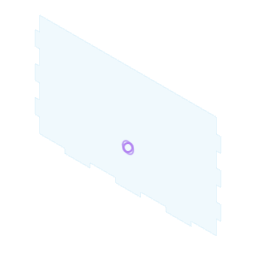
Box for nanoboard (Autodesk Fusion 360 design; units mm, degrees)
Autodesk Fusion 360 part; units mm, degrees
note: some values were not read from the file. Set by a fixed rule: which sketch regions a step uses.
(part 1 of 2)
sketch "Sketch1" plane through (0, 0, 0) normal (0, 1, 0) x (1, 0, 0) in component "Back"
  line L0 (0, 0) -> (126.286, 0)
  line L1 (126.286, 0) -> (126.286, -73)
  line L2 (126.286, -73) -> (0, -73)
  line L3 (0, -73) -> (0, 0)
  line L4 (3, -73) -> (3, 0)
  line L5 (0, -13) -> (3, -13)
  line L6 (0, -23) -> (3, -23)
  line L7 (3, -35) -> (3, -33)
  line L8 (3, -33) -> (0, -33)
  line L9 (0, -33) -> (0, -36.5)
  line L10 (0, -63) -> (3, -63)
  line L11 (3, -63) -> (3, -53)
  line L12 (3, -53) -> (0, -53)
  line L13 (0, -53) -> (0, -63)
  line L14 (0, -43) -> (3, -43)
  line L15 (63.143, -73) -> (63.143, 0) construction
  line L16 (126.286, -63) -> (123.286, -63)
  line L17 (123.286, -53) -> (126.286, -53)
  line L18 (123.286, -73) -> (123.286, 0)
  line L19 (126.286, -43) -> (123.286, -43)
  line L20 (123.286, -33) -> (126.286, -33)
  line L21 (126.286, -23) -> (123.286, -23)
  line L22 (126.286, -13) -> (123.286, -13)
  line L23 (126.286, -3) -> (0, -3)
  line L24 (106.1023, -3) -> (88.9186, -3)
  line L25 (88.9186, -3) -> (88.9186, 0)
  line L26 (88.9186, 0) -> (106.1023, 0)
  line L27 (106.1023, 0) -> (106.1023, -3)
  line L28 (71.7349, -3) -> (54.5511, -3)
  line L29 (54.5511, -3) -> (54.5511, 0)
  line L30 (54.5511, 0) -> (71.7349, 0)
  line L31 (71.7349, 0) -> (71.7349, -3)
  line L32 (37.3674, -3) -> (0, -3)
  line L33 (0, -3) -> (0, 0)
  line L34 (0, 0) -> (37.3674, 0)
  line L35 (37.3674, 0) -> (37.3674, -3)
  line L36 (126.286, -73) -> (0, -73)
  line L37 (0, -73) -> (0, -76)
  line L38 (0, -76) -> (126.286, -76)
  line L39 (126.286, -76) -> (126.286, -73)
  line L40 (123.286, -73) -> (123.286, -76)
  line L41 (3, -73) -> (3, -76)
  line L42 (20.1837, -3) -> (20.1837, 0)
  dimension "d10" = 3
  dimension "d58" = 3
  dimension "d137" = 3
  dimension "d171" = 70
  dimension "d172" = 120.286
  dimension "d173" = 17.1837
  dimension "d174" = 17.1837
  dimension "d175" = 17.1837
  dimension "d176" = 17.1837
  dimension "d177" = 17.1837
  dimension "d178" = 17.1837
  dimension "d179" = 22.8571
  dimension "d188" = 10
  dimension "d189" = 10
  dimension "d190" = 10
  dimension "d191" = 10
  dimension "d192" = 10
  dimension "d193" = 10
  dimension "d194" = 10
  constraint horizontal L0
  constraint vertical L1
  constraint horizontal L2
  constraint vertical L3
  constraint coincident L0.start L3.end
  constraint coincident L2 L4.start
  constraint coincident L0 L4.end
  constraint perpendicular L0 L4
  constraint coincident L3 L5.start
  constraint coincident L4 L5.end
  constraint perpendicular L4 L5
  constraint coincident L3 L6.start
  constraint coincident L4 L6.end
  constraint perpendicular L4 L6
  constraint vertical L7
  constraint horizontal L8
  constraint vertical L9
  constraint coincident L4 L7.end
  constraint midpoint L3 L9.end
  constraint horizontal L10
  constraint vertical L11
  constraint horizontal L12
  constraint vertical L13
  constraint coincident L4 L11.end
  constraint coincident L3 L10.start
  constraint coincident L3 L14.start
  constraint coincident L4 L14.end
  constraint perpendicular L4 L14
  constraint midpoint L2 L15.start
  constraint midpoint L0 L15.end
  constraint symmetric L4.start L15 L18.start
  constraint symmetric L4.end L15 L18.end
  constraint symmetric L5.start L15 L22.start
  constraint symmetric L5.end L15 L22.end
  constraint symmetric L6.start L15 L21.start
  constraint symmetric L6.end L15 L21.end
  constraint symmetric L7.end L15 L20.start
  constraint symmetric L8.end L15 L20.end
  constraint symmetric L10.start L15 L16.start
  constraint symmetric L10.end L15 L16.end
  constraint symmetric L11.end L15 L17.start
  constraint symmetric L12.end L15 L17.end
  constraint symmetric L14.start L15 L19.start
  constraint symmetric L14.end L15 L19.end
  constraint coincident L1 L23.start
  constraint coincident L3 L23.end
  constraint perpendicular L4 L23
  constraint horizontal L24
  constraint vertical L25
  constraint horizontal L26
  constraint vertical L27
  constraint coincident L0 L25.end
  constraint coincident L23 L24.start
  constraint horizontal L28
  constraint vertical L29
  constraint horizontal L30
  constraint vertical L31
  constraint coincident L23 L28.start
  constraint horizontal L32
  constraint vertical L33
  constraint horizontal L34
  constraint vertical L35
  constraint coincident L0 L3.end
  constraint coincident L23 L32.start
  constraint horizontal L36
  constraint vertical L37
  constraint horizontal L38
  constraint vertical L39
  constraint coincident L38 L40.end
  constraint perpendicular L36 L40
  constraint coincident L38 L41.end
  constraint perpendicular L38 L41
  constraint coincident L32 L42.start
  constraint coincident L34 L42.end
  constraint perpendicular L34 L42
  measures "d10" distance of L3 L4
  measures "d58" distance of L0 L23
  measures "d137" distance of L36 L38
  measures "d171" distance of L23 L36
  measures "d172" distance of L4 L18
  measures "d173" distance of L18 L27
  measures "d174" distance of L25 L27
  measures "d175" distance of L25 L31
  measures "d176" distance of L29 L31
  measures "d177" distance of L29 L35
  measures "d178" distance of L35 L42
  measures "d188" distance of L2 L10
  measures "d189" distance of L10 L12
  measures "d190" distance of L12 L14
  measures "d191" distance of L8 L14
  measures "d192" distance of L6 L8
  measures "d193" distance of L5 L6
  measures "d194" distance of L5 L23
extrude "Extrude1" add sketch "Sketch1" against normal blind 3 contours L0 L23 L32 L34 L35 L42 | L2 L4 L7 L11 L18 L23 L24 L28 L32 L36 | L3 L4 L5 L6 | L0 L23 L28 L29 L30 L31 | L3 L4 L7 L8 L9 L14 | L0 L23 L24 L25 L26 L27 | L3 L4 L10 L11 L12 L13 | L1 L18 L21 L22 | L2 L36 L38 L40 L41 | L1 L18 L19 L20 | L1 L16 L17 L18 makes body 1 in component "Back"
sketch "Sketch1 (2)" plane through (0, 0, 0) normal (1, 0, 0) x (0, 1, 0) in component "left"
  line L0 (0, 0) -> (-86, 0)
  line L1 (-86, 0) -> (-86, 73)
  line L2 (-86, 73) -> (0, 73)
  line L3 (0, 73) -> (0, 0)
  line L4 (0, 3) -> (-86, 3)
  line L5 (-19, 3) -> (-35, 3)
  line L6 (-35, 3) -> (-35, 0)
  line L7 (-35, 0) -> (-19, 0)
  line L8 (-19, 0) -> (-19, 3)
  line L9 (-48, 3) -> (-35, 3)
  line L10 (-43, 0) -> (-48, 0)
  line L11 (-51, 3) -> (-67, 3)
  line L12 (-67, 3) -> (-67, 0)
  line L13 (-67, 0) -> (-51, 0)
  line L14 (-51, 0) -> (-51, 3)
  line L15 (-3, 73) -> (-3, 0)
  circle A0 centre (-7.7793, 74.469) radius 5
  circle A1 centre (-7.7793, 74.469) radius 2.5
  line L16 (-43, 73) -> (-43, 0) construction
  line L17 (-83, 73) -> (-83, 0)
  line L18 (-86, 63) -> (-83, 63)
  line L19 (-83, 63) -> (-83, 31.2457)
  line L20 (-86, 31.2457) -> (-86, 63)
  line L21 (-86, 53) -> (-83, 53)
  line L22 (-83, 53) -> (-83, 43)
  line L23 (-83, 43) -> (-86, 43)
  line L24 (-86, 43) -> (-86, 53)
  line L25 (-83, 20) -> (-83, 33)
  line L26 (-83, 33) -> (-86, 33)
  line L27 (-86, 33) -> (-86, 36.5)
  line L28 (-86, 23) -> (-83, 23)
  line L29 (-83, 23) -> (-83, 13)
  line L30 (-83, 13) -> (-86, 13)
  line L31 (-86, 13) -> (-86, 23)
  line L32 (0, 63) -> (-3, 63)
  line L33 (0, 53) -> (-3, 53)
  line L34 (-3, 43) -> (0, 43)
  line L35 (-3, 33) -> (0, 33)
  line L36 (0, 23) -> (-3, 23)
  line L37 (-3, 13) -> (0, 13)
  line L38 (-86, 73) -> (0, 73)
  line L39 (0, 73) -> (0, 76)
  line L40 (0, 76) -> (-86, 76)
  line L41 (-86, 76) -> (-86, 73)
  circle A2 centre (-43, 7.9695) radius 5
  dimension "d67" = 3
  dimension "d111" = 3
  dimension "d112" = 10
  dimension "d113" = 5
  dimension "d161" = 3
  dimension "d162" = 10
  dimension "d166" = 10
  dimension "d167" = 10
  dimension "d169" = 3
  dimension "d180" = 16
  dimension "d181" = 16
  dimension "d182" = 16
  dimension "d183" = 16
  dimension "d185" = 80
  dimension "d186" = 16
  dimension "d195" = 70
  dimension "d196" = 10
  dimension "d197" = 10
  dimension "d198" = 10
  dimension "d199" = 10
  dimension "d233" = 10
  constraint horizontal L0
  constraint vertical L1
  constraint horizontal L2
  constraint vertical L3
  constraint coincident L0.start L3.end
  constraint coincident L3 L4.start
  constraint coincident L1 L4.end
  constraint perpendicular L1 L4
  constraint horizontal L5
  constraint vertical L6
  constraint horizontal L7
  constraint vertical L8
  constraint coincident L0 L6.end
  constraint coincident L4 L5.start
  constraint horizontal L9
  constraint horizontal L10
  constraint midpoint L0 L10.start
  constraint coincident L4 L9.start
  constraint horizontal L11
  constraint vertical L12
  constraint horizontal L13
  constraint vertical L14
  constraint coincident L0 L12.end
  constraint coincident L4 L11.start
  constraint coincident L2 L15.start
  constraint coincident L0 L15.end
  constraint perpendicular L0 L15
  constraint coincident L15.start A0
  constraint concentric A0 A1
  constraint midpoint L2 L16.start
  constraint coincident L2 L17.start
  constraint coincident L0 L17.end
  constraint perpendicular L0 L17
  constraint horizontal L18
  constraint vertical L19
  constraint vertical L20
  constraint coincident L17 L19.end
  constraint coincident L1 L18.start
  constraint horizontal L21
  constraint vertical L22
  constraint horizontal L23
  constraint vertical L24
  constraint coincident L17 L22.end
  constraint coincident L1 L21.start
  constraint vertical L25
  constraint horizontal L26
  constraint vertical L27
  constraint coincident L17 L25.end
  constraint midpoint L1 L27.end
  constraint horizontal L28
  constraint vertical L29
  constraint horizontal L30
  constraint vertical L31
  constraint coincident L17 L29.end
  constraint coincident L1 L28.start
  constraint symmetric L16 L18.start L32.start
  constraint symmetric L16 L18.end L32.end
  constraint symmetric L16 L21.start L33.start
  constraint symmetric L16 L21.end L33.end
  constraint symmetric L16 L22.end L34.start
  constraint symmetric L16 L23.end L34.end
  constraint symmetric L16 L25.end L35.start
  constraint symmetric L16 L26.end L35.end
  constraint symmetric L16 L28.start L36.start
  constraint symmetric L16 L28.end L36.end
  constraint symmetric L16 L29.end L37.start
  constraint symmetric L16 L30.end L37.end
  constraint horizontal L38
  constraint vertical L39
  constraint horizontal L40
  constraint vertical L41
  constraint coincident L16 A2.centre
  measures "d67" distance of L0 L4
  measures "d111" distance of L3 L15
  measures "d112" diameter of A0
  measures "d113" diameter of A1
  measures "d161" distance of L1 L17
  measures "d162" distance of L2 L18
  measures "d166" distance of L18 L21
  measures "d167" distance of L21 L23
  measures "d169" distance of L38 L40
  measures "d180" distance of L8 L15
  measures "d181" distance of L6 L8
  measures "d182" distance of L6 L14
  measures "d183" distance of L12 L14
  measures "d185" distance of L15 L17
  measures "d186" distance of L12 L17
  measures "d195" distance of L2 L4
  measures "d196" distance of L23 L26
  measures "d197" distance of L26 L28
  measures "d198" distance of L28 L30
  measures "d199" distance of L4 L30
  measures "d233" diameter of A2
extrude "Extrude1'" add sketch "Sketch1 (2)" along normal blind 3 separate body contours L3 L4 L15 L37 | L0 L4 L5 L6 L7 L8 | L2 L4 L5 L9 L11 L15 A0 L17 L19 L22 L25 L29 L38 A2 | L3 L15 L35 L36 | L3 L15 L33 L34 | L0 L4 L11 L12 L13 L14 | L2 L3 L15 L32 L38 | L1 L4 L17 L30 | L2 A0 A1 L38 | L2 A0 A1 L38 L40 | L2 A0 A1 L38 L40 | L2 A0 L38 L40 L41 | A0 A1 L40 | L1 L2 L17 L18 L38 | L1 L17 L19 L20 L25 L26 L28 | L1 L17 L19 L20 L21 L22 L23 L24 makes body 2 in component "left"
ref_plane "WorkPlane3" through (63.143, -43, 38) normal (0, 1, 0) x (1, 0, 0)
sketch "Sketch2" plane through (32.5, -43, 21.5) normal (0, 1, 0) x (1, 0, 0) in component "Front"
  line L0 (0, 0) -> (126.286, 0)
  line L1 (126.286, 0) -> (126.286, -73)
  line L2 (126.286, -73) -> (0, -73)
  line L3 (0, -73) -> (0, 0)
  line L4 (3, -73) -> (3, 0)
  line L5 (0, -3) -> (126.286, -3)
  line L6 (123.286, -73) -> (123.286, 0)
  line L7 (0, -73) -> (3, -73)
  line L8 (3, -73) -> (3, -63)
  line L9 (3, -63) -> (0, -63)
  line L10 (0, -63) -> (0, -73)
  line L11 (0, -53) -> (3, -53)
  line L12 (3, -53) -> (3, -43)
  line L13 (3, -43) -> (0, -43)
  line L14 (0, -43) -> (0, -53)
  line L15 (0, -33) -> (3, -33)
  line L16 (3, -33) -> (3, -23)
  line L17 (3, -23) -> (0, -23)
  line L18 (0, -23) -> (0, -33)
  line L19 (0, -13) -> (3, -13)
  line L20 (3, -13) -> (3, -4.1383)
  line L21 (0, -4.1383) -> (0, -13)
  line L22 (17.1837, -3) -> (18.5714, -3)
  line L23 (18.5714, 0) -> (17.1837, 0)
  line L24 (20.1837, -3) -> (37.3674, -3)
  line L25 (37.3674, -3) -> (37.3674, 0)
  line L26 (37.3674, 0) -> (20.1837, 0)
  line L27 (20.1837, 0) -> (20.1837, -3)
  line L28 (54.5511, -3) -> (71.7349, -3)
  line L29 (71.7349, -3) -> (71.7349, 0)
  line L30 (71.7349, 0) -> (54.5511, 0)
  line L31 (54.5511, 0) -> (54.5511, -3)
  line L32 (88.9186, -3) -> (106.1023, -3)
  line L33 (106.1023, -3) -> (106.1023, 0)
  line L34 (106.1023, 0) -> (88.9186, 0)
  line L35 (88.9186, 0) -> (88.9186, -3)
  line L36 (63.143, -73) -> (63.143, 0) construction
  line L37 (123.286, -63) -> (126.286, -63)
  line L38 (126.286, -53) -> (123.286, -53)
  line L39 (123.286, -43) -> (126.286, -43)
  line L40 (126.286, -33) -> (123.286, -33)
  line L41 (123.286, -23) -> (126.286, -23)
  line L42 (126.286, -13) -> (123.286, -13)
  circle A0 centre (63.15, -25) radius 3.5
  dimension "d140" = 3
  dimension "d141" = 3
  dimension "d142" = 3
  dimension "d187" = 70
  dimension "d200" = 10
  dimension "d201" = 10
  dimension "d202" = 10
  dimension "d203" = 10
  dimension "d204" = 10
  dimension "d205" = 10
  dimension "d206" = 10
  dimension "d209" = 120.286
  dimension "d224" = 17.1837
  dimension "d225" = 17.1837
  dimension "d226" = 17.1837
  dimension "d227" = 17.1837
  dimension "d228" = 17.1837
  dimension "d229" = 17.1837
  dimension "d230" = 17.1837
  dimension "d231" = 7
  constraint horizontal L0
  constraint vertical L1
  constraint horizontal L2
  constraint vertical L3
  constraint coincident L0.start L3.end
  constraint coincident L2 L4.start
  constraint coincident L0 L4.end
  constraint perpendicular L0 L4
  constraint coincident L3 L5.start
  constraint coincident L1 L5.end
  constraint perpendicular L1 L5
  constraint coincident L2 L6.start
  constraint coincident L0 L6.end
  constraint perpendicular L0 L6
  constraint horizontal L7
  constraint vertical L8
  constraint horizontal L9
  constraint vertical L10
  constraint coincident L4 L8.end
  constraint horizontal L11
  constraint vertical L12
  constraint horizontal L13
  constraint vertical L14
  constraint coincident L4 L12.end
  constraint coincident L3 L11.start
  constraint horizontal L15
  constraint vertical L16
  constraint horizontal L17
  constraint vertical L18
  constraint coincident L4 L16.end
  constraint coincident L3 L15.start
  constraint horizontal L19
  constraint vertical L20
  constraint vertical L21
  constraint coincident L4 L20.end
  constraint coincident L3 L19.start
  constraint horizontal L22
  constraint horizontal L23
  constraint coincident L0 L23.start
  constraint coincident L5 L22.start
  constraint horizontal L24
  constraint vertical L25
  constraint horizontal L26
  constraint vertical L27
  constraint coincident L0 L25.end
  constraint coincident L5 L24.start
  constraint horizontal L28
  constraint vertical L29
  constraint horizontal L30
  constraint vertical L31
  constraint coincident L0 L29.end
  constraint coincident L5 L28.start
  constraint horizontal L32
  constraint vertical L33
  constraint horizontal L34
  constraint vertical L35
  constraint coincident L0 L33.end
  constraint coincident L5 L32.start
  constraint midpoint L2 L36.start
  constraint midpoint L0 L36.end
  constraint symmetric L8.end L36 L37.start
  constraint symmetric L9.end L36 L37.end
  constraint symmetric L11.start L36 L38.start
  constraint symmetric L11.end L36 L38.end
  constraint symmetric L12.end L36 L39.start
  constraint symmetric L13.end L36 L39.end
  constraint symmetric L15.start L36 L40.start
  constraint symmetric L15.end L36 L40.end
  constraint symmetric L16.end L36 L41.start
  constraint symmetric L17.end L36 L41.end
  constraint symmetric L19.start L36 L42.start
  constraint symmetric L19.end L36 L42.end
  measures "d140" distance of L3 L4
  measures "d141" distance of L1 L6
  measures "d142" distance of L0 L5
  measures "d187" distance of L2 L5
  measures "d200" distance of L2 L9
  measures "d201" distance of L9 L11
  measures "d202" distance of L11 L13
  measures "d203" distance of L13 L15
  measures "d204" distance of L15 L17
  measures "d205" distance of L17 L19
  measures "d206" distance of L5 L19
  measures "d209" distance of L4 L6
  measures "d224" distance of L6 L33
  measures "d225" distance of L33 L35
  measures "d226" distance of L29 L35
  measures "d227" distance of L29 L31
  measures "d228" distance of L25 L31
  measures "d229" distance of L25 L27
  measures "d230" distance of L4 L27
  measures "d231" diameter of A0
extrude "Extrude1''" add sketch "Sketch2" along normal blind 3 separate body contours L2 L4 L5 L6 L8 L12 L16 L20 L22 L24 L28 L32 | L3 L4 L17 L19 | L0 L5 L24 L25 L26 L27 | L3 L4 L13 L15 | L0 L5 L28 L29 L30 L31 | L3 L4 L9 L11 | L0 L5 L32 L33 L34 L35 | L1 L6 L41 L42 | L1 L6 L37 L38 | L1 L6 L39 L40 makes body 3 in component "Front"
move_body "Move1" bodies 3 to x (1, 0, 0) y (0, 1, 0) z (0, 0, 1) at (-32.5004, -25.4546, -21.3867) in component "Front"
ref_plane "WorkPlane5" through (63.143, -43, 40.3645) normal (1, 0, 0) x (0, 1, 0)
mirror "Mirror1" about plane through (63.143, -43, 40.3645) normal (1, 0, 0) of bodies 2 makes body 4 in component "left"
move_body "Move3" bodies 3 to x (1, 0, 0) y (0, 1, 0) z (0, 0, 1) at (0.0007, 0, -0.1134) in component "Front"
sketch "Sketch1 (3)" plane through (0, 0, 0) normal (0, 0, 1) x (1, 0, 0) in component "lid"
  line L0 (0, 0) -> (126.286, 0)
  line L1 (126.286, 0) -> (126.286, -86)
  line L2 (126.286, -86) -> (0, -86)
  line L3 (0, -86) -> (0, 0)
  line L4 (3, 0) -> (3, -86)
  line L5 (0, -6) -> (3, -6)
  line L6 (3, -6) -> (3, -9)
  line L7 (3, -9) -> (0, -9)
  line L8 (0, -9) -> (0, -6)
  line L9 (63.143, 0) -> (63.143, -86) construction
  line L10 (123.286, 0) -> (123.286, -86)
  line L11 (126.286, -6) -> (123.286, -6)
  line L12 (123.286, -9) -> (126.286, -9)
  line L13 (0, -83) -> (126.286, -83)
  line L14 (0, -3) -> (126.286, -3)
  dimension "d98" = 3
  dimension "d99" = 3
  dimension "d103" = 3
  dimension "d109" = 3
  dimension "d114" = 3
  dimension "d207" = 120.286
  dimension "d208" = 80
  constraint horizontal L0
  constraint vertical L1
  constraint horizontal L2
  constraint vertical L3
  constraint coincident L0.start L3.end
  constraint coincident L0 L4.start
  constraint coincident L2 L4.end
  constraint perpendicular L2 L4
  constraint horizontal L5
  constraint vertical L6
  constraint horizontal L7
  constraint vertical L8
  constraint coincident L4 L6.end
  constraint coincident L3 L5.start
  constraint midpoint L0 L9.start
  constraint midpoint L2 L9.end
  constraint symmetric L4.start L9 L10.start
  constraint symmetric L4.end L9 L10.end
  constraint symmetric L5.start L9 L11.start
  constraint symmetric L5.end L9 L11.end
  constraint symmetric L6.end L9 L12.start
  constraint symmetric L7.end L9 L12.end
  constraint coincident L3 L13.start
  constraint coincident L1 L13.end
  constraint perpendicular L1 L13
  constraint coincident L3 L14.start
  constraint coincident L1 L14.end
  constraint perpendicular L1 L14
  measures "d98" distance of L5 L7
  measures "d99" distance of L3 L4
  measures "d103" distance of L2 L13
  measures "d109" distance of L0 L14
  measures "d114" distance of L5 L14
  measures "d207" distance of L4 L10
  measures "d208" distance of L13 L14
extrude "Extrude1'''" add sketch "Sketch1 (3)" along normal blind 3 separate body contours L4 L6 L10 L13 L14 | L3 L4 L5 L6 L7 L8 | L1 L10 L11 L12 | L2 L4 L10 L13 makes body 5 in component "lid"
move_body "Move2" bodies 5 to x (1, 0, 0) y (0, 1, 0) z (0, 0, 1) at (0, 0, 73) in component "lid"
move_body "Move4" bodies 3 to x (1, 0, 0) y (0, 1, 0) z (0, 0, 1) at (0.0064, -17, 0) in component "Front"
sketch "back_dxf" plane through (0, -3, 0) normal (0, -1, 0) x (1, 0, 0)
  line L0 (3, 76) -> (3, 63)
  line L1 (3, 63) -> (0, 63)
  line L2 (0, 63) -> (0, 53)
  line L3 (0, 53) -> (3, 53)
  line L4 (3, 53) -> (3, 43)
  line L5 (3, 43) -> (0, 43)
  line L6 (0, 43) -> (0, 33)
  line L7 (0, 33) -> (3, 33)
  line L8 (3, 33) -> (3, 23)
  line L9 (3, 23) -> (0, 23)
  line L10 (0, 23) -> (0, 13)
  line L11 (0, 13) -> (3, 13)
  line L12 (3, 13) -> (3, 3)
  line L13 (20.1837, 0) -> (37.3674, 0)
  line L14 (37.3674, 0) -> (37.3674, 3)
  line L15 (54.5511, 3) -> (54.5511, 0)
  line L16 (71.7349, 0) -> (71.7349, 3)
  line L17 (88.9186, 3) -> (88.9186, 0)
  line L18 (3, 3) -> (20.1837, 3)
  line L19 (106.1023, 0) -> (106.1023, 3)
  line L20 (123.286, 3) -> (123.286, 13)
  line L21 (123.286, 13) -> (126.286, 13)
  line L22 (126.286, 13) -> (126.286, 23)
  line L23 (126.286, 23) -> (123.286, 23)
  line L24 (123.286, 23) -> (123.286, 33)
  line L25 (123.286, 33) -> (126.286, 33)
  line L26 (126.286, 33) -> (126.286, 43)
  line L27 (126.286, 43) -> (123.286, 43)
  line L28 (123.286, 43) -> (123.286, 53)
  line L29 (123.286, 53) -> (126.286, 53)
  line L30 (126.286, 53) -> (126.286, 63)
  line L31 (126.286, 63) -> (123.286, 63)
  line L32 (123.286, 63) -> (123.286, 76)
  line L33 (123.286, 76) -> (3, 76)
  line L34 (37.3674, 3) -> (54.5511, 3)
  line L35 (54.5511, 0) -> (71.7349, 0)
  line L36 (88.9186, 0) -> (106.1023, 0)
  line L37 (106.1023, 3) -> (123.286, 3)
  line L38 (20.1837, 3) -> (20.1837, 0)
  line L39 (71.7349, 3) -> (88.9186, 3)
sketch "left_dxf" plane through (126.286, 0, 0) normal (1, 0, 0) x (0, 1, 0)
  circle A0 centre (-7.7793, 74.469) radius 2.5
  arc A1 (-3, 73) -> (-12.5392, 76) centre (-7.7793, 74.469) ccw
  line L0 (-12.5392, 76) -> (-86, 76)
  line L1 (-86, 76) -> (-86, 63)
  line L2 (-86, 63) -> (-83, 63)
  line L3 (-83, 63) -> (-83, 53)
  line L4 (-83, 53) -> (-86, 53)
  line L5 (-86, 53) -> (-86, 43)
  line L6 (-86, 43) -> (-83, 43)
  line L7 (-83, 43) -> (-83, 33)
  line L8 (-83, 33) -> (-86, 33)
  line L9 (-86, 33) -> (-86, 23)
  line L10 (-86, 23) -> (-83, 23)
  line L11 (-83, 23) -> (-83, 13)
  line L12 (-83, 13) -> (-86, 13)
  line L13 (-86, 13) -> (-86, 3)
  line L14 (-86, 3) -> (-67, 3)
  line L15 (-67, 3) -> (-67, 0)
  line L16 (-35, 0) -> (-19, 0)
  line L17 (-19, 0) -> (-19, 3)
  line L18 (-19, 3) -> (0, 3)
  line L19 (0, 3) -> (0, 13)
  line L20 (0, 13) -> (-3, 13)
  line L21 (-3, 13) -> (-3, 23)
  line L22 (-3, 23) -> (0, 23)
  line L23 (0, 23) -> (0, 33)
  line L24 (0, 33) -> (-3, 33)
  line L25 (-3, 33) -> (-3, 43)
  line L26 (-3, 43) -> (0, 43)
  line L27 (0, 43) -> (0, 53)
  line L28 (0, 53) -> (-3, 53)
  line L29 (-3, 53) -> (-3, 63)
  line L30 (-3, 63) -> (0, 63)
  line L31 (0, 63) -> (0, 73)
  line L32 (0, 73) -> (-3, 73)
  line L33 (-51, 0) -> (-51, 3)
  line L34 (-51, 3) -> (-43.5512, 3)
  line L35 (-35, 3) -> (-35, 0)
  line L36 (-67, 0) -> (-51, 0)
  arc A2 (-42.4488, 3) -> (-43.5512, 3) centre (-43, 7.9695) ccw
  line L37 (-42.4488, 3) -> (-35, 3)
sketch "front_dxf" plane through (0, -85.4546, 0) normal (0, -1, 0) x (1, 0, 0)
  line L0 (123.2928, 32.9999) -> (126.2928, 32.9999)
  line L1 (126.2928, 32.9999) -> (126.2928, 42.9999)
  line L2 (126.2928, 42.9999) -> (123.2928, 42.9999)
  line L3 (123.2928, 42.9999) -> (123.2928, 52.9999)
  line L4 (123.2928, 52.9999) -> (126.2928, 52.9999)
  line L5 (126.2928, 52.9999) -> (126.2928, 62.9999)
  line L6 (126.2928, 62.9999) -> (123.2928, 62.9999)
  line L7 (123.2928, 62.9999) -> (123.2928, 72.9999)
  line L8 (123.2928, 72.9999) -> (3.0068, 72.9999)
  line L9 (3.0068, 72.9999) -> (3.0068, 62.9999)
  line L10 (3.0068, 62.9999) -> (0.0068, 62.9999)
  line L11 (0.0068, 62.9999) -> (0.0068, 52.9999)
  line L12 (0.0068, 52.9999) -> (3.0068, 52.9999)
  line L13 (3.0068, 52.9999) -> (3.0068, 42.9999)
  line L14 (3.0068, 42.9999) -> (0.0068, 42.9999)
  line L15 (0.0068, 42.9999) -> (0.0068, 32.9999)
  line L16 (0.0068, 32.9999) -> (3.0068, 32.9999)
  line L17 (3.0068, 32.9999) -> (3.0068, 22.9999)
  line L18 (3.0068, 22.9999) -> (0.0068, 22.9999)
  line L19 (0.0068, 22.9999) -> (0.0068, 12.9999)
  line L20 (0.0068, 12.9999) -> (3.0068, 12.9999)
  line L21 (3.0068, 12.9999) -> (3.0068, 2.9999)
  line L22 (20.1905, 2.9999) -> (20.1905, -0.0001)
  line L23 (3.0068, 2.9999) -> (20.1905, 2.9999)
  line L24 (37.3742, -0.0001) -> (37.3742, 2.9999)
  line L25 (20.1905, -0.0001) -> (37.3742, -0.0001)
  line L26 (54.5579, 2.9999) -> (54.5579, -0.0001)
  line L27 (37.3742, 2.9999) -> (54.5579, 2.9999)
  line L28 (71.7416, -0.0001) -> (71.7416, 2.9999)
  line L29 (54.5579, -0.0001) -> (71.7416, -0.0001)
  line L30 (88.9253, 2.9999) -> (88.9253, -0.0001)
  line L31 (71.7416, 2.9999) -> (88.9253, 2.9999)
  line L32 (106.109, -0.0001) -> (106.109, 2.9999)
  line L33 (88.9253, -0.0001) -> (106.109, -0.0001)
  line L34 (123.2928, 2.9999) -> (123.2928, 12.9999)
  line L35 (123.2928, 12.9999) -> (126.2928, 12.9999)
  line L36 (126.2928, 12.9999) -> (126.2928, 22.9999)
  line L37 (126.2928, 22.9999) -> (123.2928, 22.9999)
  line L38 (123.2928, 22.9999) -> (123.2928, 32.9999)
  line L39 (106.109, 2.9999) -> (123.2928, 2.9999)
  circle A0 centre (63.1568, 24.9999) radius 3.5
sketch "base_dxf" plane through (0, 0, 0) normal (0, 0, -1) x (1, 0, 0)
  line L0 (23.1841, 65.4546) -> (23.1841, 68.4546)
  line L1 (40.3678, 65.4546) -> (23.1841, 65.4546)
  line L2 (23.1841, 68.4546) -> (40.3678, 68.4546)
  line L3 (57.5515, 65.4546) -> (57.5515, 68.4546)
  line L4 (40.3678, 68.4546) -> (40.3678, 65.4546)
  line L5 (91.9189, 65.4546) -> (91.9189, 68.4546)
  line L6 (74.7352, 68.4546) -> (74.7352, 65.4546)
  line L7 (109.1026, 68.4546) -> (109.1026, 65.4546)
  line L8 (3, 19) -> (0, 19)
  line L9 (0, 19) -> (0, 35)
  line L10 (0, 67) -> (3, 67)
  line L11 (3, 35) -> (3, 19)
  line L12 (106.1023, 3) -> (106.1023, 0)
  line L13 (88.9186, 3) -> (106.1023, 3)
  line L14 (106.1023, 0) -> (88.9186, 0)
  line L15 (71.7349, 3) -> (71.7349, 0)
  line L16 (88.9186, 0) -> (88.9186, 3)
  line L17 (37.3674, 3) -> (37.3674, 0)
  line L18 (54.5511, 0) -> (54.5511, 3)
  line L19 (-3, -3) -> (123.286, -3)
  line L20 (123.286, -3) -> (123.286, 83)
  line L21 (123.286, 83) -> (-3, 83)
  line L22 (-3, 83) -> (-3, -3)
  line L23 (3, 51) -> (0, 51)
  line L24 (0, 51) -> (0, 67)
  line L25 (54.5511, 3) -> (71.7349, 3)
  line L26 (71.7349, 0) -> (54.5511, 0)
  line L27 (37.3674, 0) -> (20.1837, 0)
  line L28 (74.7352, 65.4546) -> (57.5515, 65.4546)
  line L29 (57.5515, 68.4546) -> (74.7352, 68.4546)
  line L30 (109.1026, 65.4546) -> (91.9189, 65.4546)
  line L31 (91.9189, 68.4546) -> (109.1026, 68.4546)
  line L32 (20.1837, 0) -> (20.1837, 3)
  line L33 (20.1837, 3) -> (37.3674, 3)
  line L34 (0, 35) -> (3, 35)
  line L35 (3, 67) -> (3, 51)
sketch "lid_dxf" plane through (0, 0, 73) normal (0, 0, -1) x (1, 0, 0)
  line L0 (3, 3) -> (123.286, 3)
  line L1 (123.286, 3) -> (123.286, 6)
  line L2 (123.286, 6) -> (126.286, 6)
  line L3 (126.286, 6) -> (126.286, 9)
  line L4 (126.286, 9) -> (123.286, 9)
  line L5 (123.286, 9) -> (123.286, 86)
  line L6 (123.286, 86) -> (3, 86)
  line L7 (3, 86) -> (3, 9)
  line L8 (3, 9) -> (0, 9)
  line L9 (0, 9) -> (0, 6)
  line L10 (0, 6) -> (3, 6)
  line L11 (3, 6) -> (3, 3)
sketch "left big_dxf" plane through (126.286, 0, 0) normal (1, 0, 0) x (0, 1, 0)
  line L0 (-12.5392, 76) -> (-86, 76)
  line L1 (-86, 76) -> (-86, 63)
  line L2 (-86, 63) -> (-83, 63)
  line L3 (-83, 63) -> (-83, 53)
  line L4 (-83, 53) -> (-86, 53)
  line L5 (-86, 53) -> (-86, 43)
  line L6 (-86, 43) -> (-83, 43)
  line L7 (-83, 43) -> (-83, 33)
  line L8 (-83, 33) -> (-86, 33)
  line L9 (-86, 33) -> (-86, 23)
  line L10 (-86, 23) -> (-83, 23)
  line L11 (-83, 23) -> (-83, 13)
  line L12 (-83, 13) -> (-86, 13)
  line L13 (-86, 13) -> (-86, 3)
  line L14 (-86, 3) -> (-67, 3)
  line L15 (-67, 3) -> (-67, 0)
  line L16 (-35, 0) -> (-19, 0)
  line L17 (-19, 0) -> (-19, 3)
  line L18 (-19, 3) -> (0, 3)
  line L19 (0, 3) -> (0, 13)
  line L20 (0, 13) -> (-3, 13)
  line L21 (-3, 13) -> (-3, 23)
  line L22 (-3, 23) -> (0, 23)
  line L23 (0, 23) -> (0, 33)
  line L24 (0, 33) -> (-3, 33)
  line L25 (-3, 33) -> (-3, 43)
  line L26 (-3, 43) -> (0, 43)
  line L27 (0, 43) -> (0, 53)
  line L28 (0, 53) -> (-3, 53)
  line L29 (-3, 53) -> (-3, 63)
  line L30 (-3, 63) -> (0, 63)
  line L31 (0, 63) -> (0, 73)
  line L32 (0, 73) -> (-3, 73)
  arc A0 (-3, 73) -> (-12.5392, 76) centre (-7.7793, 74.469) ccw
  circle A1 centre (-7.7793, 74.469) radius 2.5
  line L33 (-51, 0) -> (-51, 3)
  line L34 (-51, 3) -> (-43.5512, 3)
  line L35 (-35, 3) -> (-35, 0)
  line L36 (-67, 0) -> (-51, 0)
  arc A2 (-42.4488, 3) -> (-43.5512, 3) centre (-43, 7.9695) ccw
  line L37 (-42.4488, 3) -> (-35, 3)
sketch "final" plane through (0, 0, 76) normal (0, 0, 1) x (-1, 0, 0) in component "lid"
  line L0 (-123.286, 3) -> (-3, 3)
  line L1 (-3, 3) -> (-3, 6)
  line L2 (-3, 6) -> (0, 6)
  line L3 (0, 6) -> (0, 9)
  line L4 (0, 9) -> (-3, 9)
  line L5 (-3, 9) -> (-3, 86)
  line L6 (-3, 86) -> (-123.286, 86)
  line L7 (-123.286, 86) -> (-123.286, 9)
  line L8 (-123.286, 9) -> (-126.286, 9)
  line L9 (-126.286, 9) -> (-126.286, 6)
  line L10 (-126.286, 6) -> (-123.286, 6)
  line L11 (-123.286, 6) -> (-123.286, 3)
sketch "final (2)" plane through (0, -85.4546, 0) normal (0, -1, 0) x (1, 0, 0) in component "Front"
  line L0 (54.5579, 2.9999) -> (54.5579, -0.0001)
  line L1 (37.3742, 2.9999) -> (54.5579, 2.9999)
  line L2 (71.7416, -0.0001) -> (71.7416, 2.9999)
  line L3 (54.5579, -0.0001) -> (71.7416, -0.0001)
  line L4 (88.9253, 2.9999) -> (88.9253, -0.0001)
  line L5 (71.7416, 2.9999) -> (88.9253, 2.9999)
  line L6 (106.109, -0.0001) -> (106.109, 2.9999)
  line L7 (88.9253, -0.0001) -> (106.109, -0.0001)
  line L8 (123.2928, 2.9999) -> (123.2928, 12.9999)
  line L9 (123.2928, 12.9999) -> (126.2928, 12.9999)
  line L10 (126.2928, 12.9999) -> (126.2928, 22.9999)
  line L11 (126.2928, 22.9999) -> (123.2928, 22.9999)
  line L12 (123.2928, 22.9999) -> (123.2928, 32.9999)
  line L13 (123.2928, 32.9999) -> (126.2928, 32.9999)
  line L14 (126.2928, 32.9999) -> (126.2928, 42.9999)
  line L15 (126.2928, 42.9999) -> (123.2928, 42.9999)
  line L16 (123.2928, 42.9999) -> (123.2928, 52.9999)
  line L17 (123.2928, 52.9999) -> (126.2928, 52.9999)
  line L18 (126.2928, 52.9999) -> (126.2928, 62.9999)
  line L19 (126.2928, 62.9999) -> (123.2928, 62.9999)
  line L20 (123.2928, 62.9999) -> (123.2928, 72.9999)
  line L21 (123.2928, 72.9999) -> (3.0068, 72.9999)
  line L22 (3.0068, 72.9999) -> (3.0068, 62.9999)
  line L23 (3.0068, 62.9999) -> (0.0068, 62.9999)
  line L24 (0.0068, 62.9999) -> (0.0068, 52.9999)
  line L25 (0.0068, 52.9999) -> (3.0068, 52.9999)
  line L26 (3.0068, 52.9999) -> (3.0068, 42.9999)
  line L27 (3.0068, 42.9999) -> (0.0068, 42.9999)
  line L28 (0.0068, 42.9999) -> (0.0068, 32.9999)
  line L29 (0.0068, 32.9999) -> (3.0068, 32.9999)
  line L30 (3.0068, 32.9999) -> (3.0068, 22.9999)
  line L31 (3.0068, 22.9999) -> (0.0068, 22.9999)
  line L32 (0.0068, 22.9999) -> (0.0068, 12.9999)
  line L33 (0.0068, 12.9999) -> (3.0068, 12.9999)
  line L34 (3.0068, 12.9999) -> (3.0068, 2.9999)
  line L35 (20.1905, 2.9999) -> (20.1905, -0.0001)
  line L36 (3.0068, 2.9999) -> (20.1905, 2.9999)
  line L37 (37.3742, -0.0001) -> (37.3742, 2.9999)
  line L38 (20.1905, -0.0001) -> (37.3742, -0.0001)
  line L39 (106.109, 2.9999) -> (123.2928, 2.9999)
  circle A0 centre (63.1568, 24.9999) radius 3.5
sketch "Sketch4" plane through (0, -82.4546, 0) normal (0, 1, 0) x (-1, 0, 0) in component "Front"
  line L0 (-126.2928, 32.9999) -> (-123.2928, 32.9999)
  line L1 (-123.2928, 32.9999) -> (-123.2928, 22.9999)
  line L2 (-123.2928, 22.9999) -> (-126.2928, 22.9999)
  line L3 (-126.2928, 22.9999) -> (-126.2928, 12.9999)
  line L4 (-126.2928, 12.9999) -> (-123.2928, 12.9999)
  line L5 (-123.2928, 12.9999) -> (-123.2928, 2.9999)
  line L6 (-123.2928, 2.9999) -> (-106.109, 2.9999)
  line L7 (-106.109, 2.9999) -> (-106.109, -0.0001)
  line L8 (-106.109, -0.0001) -> (-88.9253, -0.0001)
  line L9 (-88.9253, -0.0001) -> (-88.9253, 2.9999)
  line L10 (-88.9253, 2.9999) -> (-71.7416, 2.9999)
  line L11 (-71.7416, 2.9999) -> (-71.7416, -0.0001)
  line L12 (-71.7416, -0.0001) -> (-54.5579, -0.0001)
  line L13 (-54.5579, -0.0001) -> (-54.5579, 2.9999)
  line L14 (-54.5579, 2.9999) -> (-37.3742, 2.9999)
  line L15 (-37.3742, 2.9999) -> (-37.3742, -0.0001)
  line L16 (-37.3742, -0.0001) -> (-20.1905, -0.0001)
  line L17 (-20.1905, -0.0001) -> (-20.1905, 2.9999)
  line L18 (-20.1905, 2.9999) -> (-3.0068, 2.9999)
  line L19 (-3.0068, 2.9999) -> (-3.0068, 12.9999)
  line L20 (-3.0068, 12.9999) -> (-0.0068, 12.9999)
  line L21 (-0.0068, 12.9999) -> (-0.0068, 22.9999)
  line L22 (-0.0068, 22.9999) -> (-3.0068, 22.9999)
  line L23 (-3.0068, 22.9999) -> (-3.0068, 32.9999)
  line L24 (-3.0068, 32.9999) -> (-0.0068, 32.9999)
  line L25 (-0.0068, 32.9999) -> (-0.0068, 42.9999)
  line L26 (-0.0068, 42.9999) -> (-3.0068, 42.9999)
  line L27 (-3.0068, 42.9999) -> (-3.0068, 52.9999)
  line L28 (-3.0068, 52.9999) -> (-0.0068, 52.9999)
  line L29 (-0.0068, 52.9999) -> (-0.0068, 62.9999)
  line L30 (-0.0068, 62.9999) -> (-3.0068, 62.9999)
  line L31 (-3.0068, 62.9999) -> (-3.0068, 72.9999)
  line L32 (-3.0068, 72.9999) -> (-123.2928, 72.9999)
  line L33 (-123.2928, 72.9999) -> (-123.2928, 62.9999)
  line L34 (-123.2928, 62.9999) -> (-126.2928, 62.9999)
  line L35 (-126.2928, 62.9999) -> (-126.2928, 52.9999)
  line L36 (-126.2928, 52.9999) -> (-123.2928, 52.9999)
  line L37 (-123.2928, 52.9999) -> (-123.2928, 42.9999)
  line L38 (-123.2928, 42.9999) -> (-126.2928, 42.9999)
  line L39 (-126.2928, 42.9999) -> (-126.2928, 32.9999)
  circle A0 centre (-63.1568, 24.9999) radius 3.5
sketch "Sketch2 (2)" plane through (126.286, 0, 0) normal (1, 0, 0) x (0, 1, 0) in component "left"
  circle A0 centre (-7.7793, 74.469) radius 2.5
  arc A1 (-3, 73) -> (-12.5392, 76) centre (-7.7793, 74.469) ccw
  line L0 (-12.5392, 76) -> (-86, 76)
  line L1 (-86, 76) -> (-86, 63)
  line L2 (-86, 63) -> (-83, 63)
  line L3 (-83, 63) -> (-83, 53)
  line L4 (-83, 53) -> (-86, 53)
  line L5 (-86, 53) -> (-86, 43)
  line L6 (-86, 43) -> (-83, 43)
  line L7 (-83, 43) -> (-83, 33)
  line L8 (-83, 33) -> (-86, 33)
  line L9 (-86, 33) -> (-86, 23)
  line L10 (-86, 23) -> (-83, 23)
  line L11 (-83, 23) -> (-83, 13)
  line L12 (-83, 13) -> (-86, 13)
  line L13 (-86, 13) -> (-86, 3)
  line L14 (-86, 3) -> (-67, 3)
  line L15 (-67, 3) -> (-67, 0)
  line L16 (-67, 0) -> (-51, 0)
  line L17 (-51, 0) -> (-51, 3)
  line L18 (-51, 3) -> (-43.5512, 3)
  line L19 (-19, 0) -> (-19, 3)
  line L20 (-19, 3) -> (0, 3)
  line L21 (0, 3) -> (0, 13)
  line L22 (0, 13) -> (-3, 13)
  line L23 (-3, 13) -> (-3, 23)
  line L24 (-3, 23) -> (0, 23)
  line L25 (0, 23) -> (0, 33)
  line L26 (0, 33) -> (-3, 33)
  line L27 (-3, 33) -> (-3, 43)
  line L28 (-3, 43) -> (0, 43)
  line L29 (0, 43) -> (0, 53)
  line L30 (0, 53) -> (-3, 53)
  line L31 (-3, 53) -> (-3, 63)
  line L32 (-3, 63) -> (0, 63)
  line L33 (0, 63) -> (0, 73)
  line L34 (0, 73) -> (-3, 73)
  line L35 (-35, 3) -> (-35, 0)
  line L36 (-35, 0) -> (-19, 0)
  arc A2 (-42.4488, 3) -> (-43.5512, 3) centre (-43, 7.9695) ccw
  line L37 (-42.4488, 3) -> (-35, 3)
sketch "Sketch4 (2)" plane through (0, -3, 0) normal (0, -1, 0) x (1, 0, 0) in component "Back"
  line L0 (0, 53) -> (3, 53)
  line L1 (3, 53) -> (3, 43)
  line L2 (3, 43) -> (0, 43)
  line L3 (0, 43) -> (0, 33)
  line L4 (0, 33) -> (3, 33)
  line L5 (3, 33) -> (3, 23)
  line L6 (3, 23) -> (0, 23)
  line L7 (0, 23) -> (0, 13)
  line L8 (0, 13) -> (3, 13)
  line L9 (3, 13) -> (3, 3)
  line L10 (20.1837, 0) -> (37.3674, 0)
  line L11 (37.3674, 0) -> (37.3674, 3)
  line L12 (37.3674, 3) -> (54.5511, 3)
  line L13 (54.5511, 3) -> (54.5511, 0)
  line L14 (54.5511, 0) -> (71.7349, 0)
  line L15 (71.7349, 0) -> (71.7349, 3)
  line L16 (3, 3) -> (20.1837, 3)
  line L17 (88.9186, 3) -> (88.9186, 0)
  line L18 (88.9186, 0) -> (106.1023, 0)
  line L19 (106.1023, 0) -> (106.1023, 3)
  line L20 (106.1023, 3) -> (123.286, 3)
  line L21 (123.286, 3) -> (123.286, 13)
  line L22 (123.286, 13) -> (126.286, 13)
  line L23 (126.286, 13) -> (126.286, 23)
  line L24 (126.286, 23) -> (123.286, 23)
  line L25 (123.286, 23) -> (123.286, 33)
  line L26 (123.286, 33) -> (126.286, 33)
  line L27 (126.286, 33) -> (126.286, 43)
  line L28 (126.286, 43) -> (123.286, 43)
  line L29 (123.286, 43) -> (123.286, 53)
  line L30 (123.286, 53) -> (126.286, 53)
  line L31 (126.286, 53) -> (126.286, 63)
  line L32 (126.286, 63) -> (123.286, 63)
  line L33 (123.286, 63) -> (123.286, 76)
  line L34 (123.286, 76) -> (3, 76)
  line L35 (3, 76) -> (3, 63)
  line L36 (3, 63) -> (0, 63)
  line L37 (0, 63) -> (0, 53)
  line L38 (20.1837, 3) -> (20.1837, 0)
  line L39 (71.7349, 3) -> (88.9186, 3)
sketch "Sketch24" plane through (63.143, -3, 38) normal (0, -1, 0) x (1, 0, 0)
sketch "Sketch25" plane through (0, 0, 0) normal (-1, 0, 0) x (0, -1, 0)
  line L0 (86, 76) -> (12.5392, 76)
  arc A0 (12.5392, 76) -> (3, 73) centre (7.7793, 74.469) ccw
  line L1 (3, 73) -> (0, 73)
  line L2 (0, 73) -> (0, 63)
  line L3 (0, 63) -> (3, 63)
  line L4 (3, 63) -> (3, 53)
  line L5 (3, 53) -> (0, 53)
  line L6 (0, 53) -> (0, 43)
  line L7 (0, 43) -> (3, 43)
  line L8 (3, 43) -> (3, 33)
  line L9 (3, 33) -> (0, 33)
  line L10 (0, 33) -> (0, 23)
  line L11 (0, 23) -> (3, 23)
  line L12 (3, 23) -> (3, 13)
  line L13 (3, 13) -> (0, 13)
  line L14 (0, 13) -> (0, 3)
  line L15 (0, 3) -> (19, 3)
  line L16 (19, 3) -> (19, 0)
  line L17 (19, 0) -> (35, 0)
  line L18 (35, 0) -> (35, 3)
  line L19 (43.5512, 3) -> (51, 3)
  line L20 (51, 3) -> (51, 0)
  line L21 (51, 0) -> (67, 0)
  line L22 (67, 0) -> (67, 3)
  line L23 (67, 3) -> (86, 3)
  line L24 (86, 3) -> (86, 13)
  line L25 (86, 13) -> (83, 13)
  line L26 (83, 13) -> (83, 23)
  line L27 (83, 23) -> (86, 23)
  line L28 (86, 23) -> (86, 33)
  line L29 (86, 33) -> (83, 33)
  line L30 (83, 33) -> (83, 43)
  line L31 (83, 43) -> (86, 43)
  line L32 (86, 43) -> (86, 53)
  line L33 (86, 53) -> (83, 53)
  line L34 (83, 53) -> (83, 63)
  line L35 (83, 63) -> (86, 63)
  line L36 (86, 63) -> (86, 76)
  circle A1 centre (7.7793, 74.469) radius 2.5
  arc A2 (43.5512, 3) -> (42.4488, 3) centre (43, 7.9695) ccw
  line L37 (35, 3) -> (42.4488, 3)
sketch "Sketch26" plane through (60.1498, -85.4546, 36.4999) normal (0, -1, 0) x (1, 0, 0)
sketch "Sketch3" plane through (0, 0, 76) normal (0, 0, 1) x (1, 0, 0) in component "lid"
sketch "Sketch4 (3)" plane through (0, 0, 76) normal (0, 0, 1) x (1, 0, 0) in component "lid"
sketch "Sketch5" plane through (0, 0, 76) normal (0, 0, 1) x (1, 0, 0) in component "lid"
sketch "Sketch27" plane through (0, 0, 3) normal (0, 0, -1) x (1, 0, 0)
  line L0 (37.3674, 0) -> (54.5511, 0)
  line L1 (54.5511, 0) -> (54.5511, 3)
  line L2 (54.5511, 3) -> (37.3674, 3)
  line L3 (37.3674, 3) -> (37.3674, 0)
  line L4 (0, 0) -> (175, 0)
  line L5 (175, 0) -> (175, 86)
  line L6 (175, 86) -> (0, 86)
  line L7 (0, 86) -> (0, 0)
  line L8 (0, 0) -> (-25, 0)
  line L9 (-25, 0) -> (-25, 86)
  line L10 (-25, 86) -> (0, 86)
  line L11 (0, 86) -> (0, 0)
  line L12 (175, 86) -> (-25, 86)
  line L13 (-25, 86) -> (-25, 96)
  line L14 (-25, 96) -> (175, 96)
  line L15 (175, 96) -> (175, 86)
  line L16 (175, 0) -> (-25, 0)
  line L17 (-25, 0) -> (-25, -10)
  line L18 (-25, -10) -> (175, -10)
  line L19 (175, -10) -> (175, 0)
  point P0 (0, 86)
  dimension "d212" = 175
  dimension "d213" = 86
  dimension "d214" = 25
  dimension "d215" = 10
  dimension "d216" = 10
  constraint horizontal L4
  constraint vertical L5
  constraint horizontal L6
  constraint vertical L7
  constraint coincident L4.start L7.end
  constraint horizontal L8
  constraint vertical L9
  constraint horizontal L10
  constraint vertical L11
  constraint coincident L10 P0
  constraint horizontal L12
  constraint vertical L13
  constraint horizontal L14
  constraint vertical L15
  constraint horizontal L16
  constraint vertical L17
  constraint horizontal L18
  constraint vertical L19
  constraint coincident L8.end L9.start
  constraint coincident L9.end L10.start
  measures "d212" distance of L4.start L5
  measures "d213" distance of L4.start P0
  measures "d214" distance of L4.start L8.end
  measures "d215" distance of L9.end L13.end
  measures "d216" distance of L8.end L17.end
extrude "Extrude1''''" add sketch "Sketch27" along normal blind 3 separate body makes body 6 in component "Top Base"
combine "Combine1" operation cut target body 6 tool bodies 1 2 4 3 keep tools in component "Top Base"
sketch "Sketch28" plane through (0, 0, 3) normal (0, 0, 1) x (-1, 0, 0)
  line L0 (-123.2928, 82.4546) -> (-123.2928, 85.4546)
  line L1 (-123.2928, 85.4546) -> (-3.0068, 85.4546)
  line L2 (-3.0068, 85.4546) -> (-3.0068, 82.4546)
  line L3 (-3.0068, 82.4546) -> (-123.2928, 82.4546)
  line L4 (-123.286, 19) -> (-126.286, 19)
  line L5 (-126.286, 19) -> (-126.286, 35)
  line L6 (-126.286, 35) -> (-123.286, 35)
  line L7 (-123.286, 35) -> (-123.286, 19)
  line L8 (-123.286, 51) -> (-126.286, 51)
  line L9 (-126.286, 51) -> (-126.286, 67)
  line L10 (-126.286, 67) -> (-123.286, 67)
  line L11 (-123.286, 67) -> (-123.286, 51)
  line L12 (0, 19) -> (-3, 19)
  line L13 (-3, 19) -> (-3, 35)
  line L14 (-3, 35) -> (0, 35)
  line L15 (0, 35) -> (0, 19)
  line L16 (0, 51) -> (-3, 51)
  line L17 (-3, 51) -> (-3, 67)
  line L18 (-3, 67) -> (0, 67)
  line L19 (0, 67) -> (0, 51)
  line L20 (-106.1023, 0) -> (-106.1023, 3)
  line L21 (-106.1023, 3) -> (-88.9186, 3)
  line L22 (-88.9186, 3) -> (-88.9186, 0)
  line L23 (-88.9186, 0) -> (-106.1023, 0)
  line L24 (-71.7349, 0) -> (-71.7349, 3)
  line L25 (-71.7349, 3) -> (-54.5511, 3)
  line L26 (-54.5511, 3) -> (-54.5511, 0)
  line L27 (-54.5511, 0) -> (-71.7349, 0)
  line L28 (-37.3674, 0) -> (-37.3674, 3)
  line L29 (-37.3674, 3) -> (-20.1837, 3)
  line L30 (-20.1837, 3) -> (-20.1837, 0)
  line L31 (-20.1837, 0) -> (-37.3674, 0)
  line L32 (25, -10) -> (25, 96)
  line L33 (25, 96) -> (-175, 96)
  line L34 (-175, 96) -> (-175, -10)
  line L35 (-175, -10) -> (25, -10)
  line L36 (-149.286, 3) -> (-146.286, 3)
  line L37 (-146.286, 3) -> (-146.286, 83)
  line L38 (-146.286, 83) -> (-149.286, 83)
  line L39 (-149.286, 83) -> (-149.286, 3)
  line L40 (-175, 43) -> (-123.572, 43) construction
  dimension "d219" = 3
  dimension "d220" = 80
  dimension "d221" = 20
  constraint horizontal L36
  constraint vertical L37
  constraint horizontal L38
  constraint vertical L39
  constraint perpendicular L34 L40
  constraint midpoint L34 L40.start
  constraint midpoint L39 L40
  measures "d219" distance of L37 L39
  measures "d220" distance of L36.start L38.end
  measures "d221" distance of L9 L37
extrude "Extrude2" cut sketch "Sketch28" against normal blind 3 contours L36 L37 L38 L39 bodies 6 in component "Top Base"
sketch "final (3)" plane through (0, -3, 0) normal (0, -1, 0) x (1, 0, 0) in component "Back"
  line L0 (3, 23) -> (0, 23)
  line L1 (0, 23) -> (0, 13)
  line L2 (0, 13) -> (3, 13)
  line L3 (3, 13) -> (3, 3)
  line L4 (3, 3) -> (20.1837, 3)
  line L5 (20.1837, 3) -> (20.1837, 0)
  line L6 (20.1837, 0) -> (37.3674, 0)
  line L7 (37.3674, 0) -> (37.3674, 3)
  line L8 (37.3674, 3) -> (54.5511, 3)
  line L9 (54.5511, 3) -> (54.5511, 0)
  line L10 (54.5511, 0) -> (71.7349, 0)
  line L11 (71.7349, 0) -> (71.7349, 3)
  line L12 (71.7349, 3) -> (88.9186, 3)
  line L13 (88.9186, 3) -> (88.9186, 0)
  line L14 (88.9186, 0) -> (106.1023, 0)
  line L15 (106.1023, 0) -> (106.1023, 3)
  line L16 (106.1023, 3) -> (123.286, 3)
  line L17 (123.286, 3) -> (123.286, 13)
  line L18 (123.286, 13) -> (126.286, 13)
  line L19 (126.286, 13) -> (126.286, 23)
  line L20 (126.286, 23) -> (123.286, 23)
  line L21 (123.286, 23) -> (123.286, 33)
  line L22 (123.286, 33) -> (126.286, 33)
  line L23 (126.286, 33) -> (126.286, 43)
  line L24 (126.286, 43) -> (123.286, 43)
  line L25 (123.286, 43) -> (123.286, 53)
  line L26 (123.286, 53) -> (126.286, 53)
  line L27 (126.286, 53) -> (126.286, 63)
  line L28 (126.286, 63) -> (123.286, 63)
  line L29 (123.286, 63) -> (123.286, 76)
  line L30 (123.286, 76) -> (3, 76)
  line L31 (3, 76) -> (3, 63)
  line L32 (3, 63) -> (0, 63)
  line L33 (0, 63) -> (0, 53)
  line L34 (0, 53) -> (3, 53)
  line L35 (3, 53) -> (3, 43)
  line L36 (3, 43) -> (0, 43)
  line L37 (0, 43) -> (0, 33)
  line L38 (0, 33) -> (3, 33)
  line L39 (3, 33) -> (3, 23)
sketch "final (4)" plane through (0, 0, 0) normal (-1, 0, 0) x (0, -1, 0) in component "left"
  line L0 (86, 76) -> (12.5392, 76)
  arc A0 (12.5392, 76) -> (3, 73) centre (7.7793, 74.469) ccw
  line L1 (3, 73) -> (0, 73)
  line L2 (0, 73) -> (0, 63)
  line L3 (0, 63) -> (3, 63)
  line L4 (3, 63) -> (3, 53)
  line L5 (3, 53) -> (0, 53)
  line L6 (0, 53) -> (0, 43)
  line L7 (0, 43) -> (3, 43)
  line L8 (3, 43) -> (3, 33)
  line L9 (3, 33) -> (0, 33)
  line L10 (0, 33) -> (0, 23)
  line L11 (0, 23) -> (3, 23)
  line L12 (3, 23) -> (3, 13)
  line L13 (3, 13) -> (0, 13)
  line L14 (0, 13) -> (0, 3)
  line L15 (0, 3) -> (19, 3)
  line L16 (19, 3) -> (19, 0)
  line L17 (19, 0) -> (35, 0)
  line L18 (35, 0) -> (35, 3)
  line L19 (43.5512, 3) -> (51, 3)
  line L20 (51, 3) -> (51, 0)
  line L21 (51, 0) -> (67, 0)
  line L22 (67, 0) -> (67, 3)
  line L23 (67, 3) -> (86, 3)
  line L24 (86, 3) -> (86, 13)
  line L25 (86, 13) -> (83, 13)
  line L26 (83, 13) -> (83, 23)
  line L27 (83, 23) -> (86, 23)
  line L28 (86, 23) -> (86, 33)
  line L29 (86, 33) -> (83, 33)
  line L30 (83, 33) -> (83, 43)
  line L31 (83, 43) -> (86, 43)
  line L32 (86, 43) -> (86, 53)
  line L33 (86, 53) -> (83, 53)
  line L34 (83, 53) -> (83, 63)
  line L35 (83, 63) -> (86, 63)
  line L36 (86, 63) -> (86, 76)
  circle A1 centre (7.7793, 74.469) radius 2.5
  arc A2 (43.5512, 3) -> (42.4488, 3) centre (43, 7.9695) ccw
  line L37 (35, 3) -> (42.4488, 3)
sketch "Sketch5 (2)" plane through (0, -85.4546, 0) normal (0, -1, 0) x (1, 0, 0) in component "Front"
  line L0 (0.0068, 52.9999) -> (3.0068, 52.9999)
  line L1 (3.0068, 52.9999) -> (3.0068, 42.9999)
  line L2 (3.0068, 42.9999) -> (0.0068, 42.9999)
  line L3 (0.0068, 42.9999) -> (0.0068, 32.9999)
  line L4 (0.0068, 32.9999) -> (3.0068, 32.9999)
  line L5 (3.0068, 32.9999) -> (3.0068, 22.9999)
  line L6 (3.0068, 22.9999) -> (0.0068, 22.9999)
  line L7 (0.0068, 22.9999) -> (0.0068, 12.9999)
  line L8 (0.0068, 12.9999) -> (3.0068, 12.9999)
  line L9 (3.0068, 12.9999) -> (3.0068, 2.9999)
  line L10 (3.0068, 2.9999) -> (20.1905, 2.9999)
  line L11 (20.1905, 2.9999) -> (20.1905, -0.0001)
  line L12 (20.1905, -0.0001) -> (37.3742, -0.0001)
  line L13 (37.3742, -0.0001) -> (37.3742, 2.9999)
  line L14 (37.3742, 2.9999) -> (54.5579, 2.9999)
  line L15 (54.5579, 2.9999) -> (54.5579, -0.0001)
  line L16 (54.5579, -0.0001) -> (71.7416, -0.0001)
  line L17 (71.7416, -0.0001) -> (71.7416, 2.9999)
  line L18 (71.7416, 2.9999) -> (88.9253, 2.9999)
  line L19 (88.9253, 2.9999) -> (88.9253, -0.0001)
  line L20 (88.9253, -0.0001) -> (106.109, -0.0001)
  line L21 (106.109, -0.0001) -> (106.109, 2.9999)
  line L22 (106.109, 2.9999) -> (123.2928, 2.9999)
  line L23 (123.2928, 2.9999) -> (123.2928, 12.9999)
  line L24 (123.2928, 12.9999) -> (126.2928, 12.9999)
  line L25 (126.2928, 12.9999) -> (126.2928, 22.9999)
  line L26 (126.2928, 22.9999) -> (123.2928, 22.9999)
  line L27 (123.2928, 22.9999) -> (123.2928, 32.9999)
  line L28 (123.2928, 32.9999) -> (126.2928, 32.9999)
  line L29 (126.2928, 32.9999) -> (126.2928, 42.9999)
  line L30 (126.2928, 42.9999) -> (123.2928, 42.9999)
  line L31 (123.2928, 42.9999) -> (123.2928, 52.9999)
  line L32 (123.2928, 52.9999) -> (126.2928, 52.9999)
  line L33 (126.2928, 52.9999) -> (126.2928, 62.9999)
  line L34 (126.2928, 62.9999) -> (123.2928, 62.9999)
  line L35 (123.2928, 62.9999) -> (123.2928, 72.9999)
  line L36 (123.2928, 72.9999) -> (3.0068, 72.9999)
  line L37 (3.0068, 72.9999) -> (3.0068, 62.9999)
  line L38 (3.0068, 62.9999) -> (0.0068, 62.9999)
  line L39 (0.0068, 62.9999) -> (0.0068, 52.9999)
  circle A0 centre (63.1568, 24.9999) radius 3.5
sketch "Sketch6" plane through (0, 0, 76) normal (0, 0, 1) x (1, 0, 0) in component "lid"